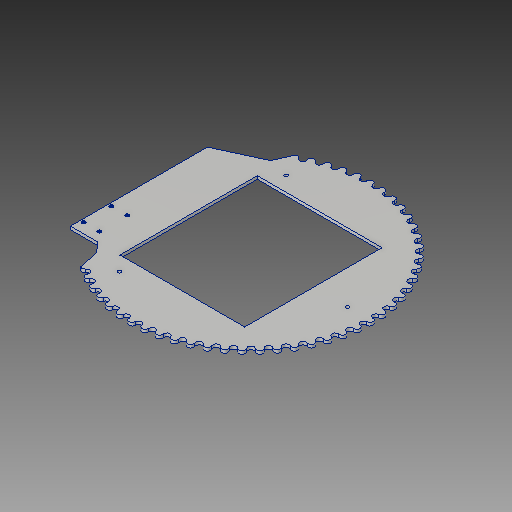
# Autodesk Inventor part: Bearing Plate
Saved by Autodesk Inventor 2019.4 (Build 234330000, 330)
## iProperties
Created: 2020-01-22
Part Number: Bearing Plate
Material: Aluminum 6061
Document SubType Name: Modeling
Designer: admin
Density: 2.7 g/cm^3
Appearance: Aluminum - Flat
Mass: 789.639 g
Surface Area: 1277.98 cm^2
Volume: 292.459 cm^3
Author: admin
Autodesk Inventor part; units mm, degrees
ref_plane "YZ Plane" through (0, 0, 0) normal (1, 0, 0) x (0, 1, 0)
ref_plane "XZ Plane" through (0, 0, 0) normal (0, 1, 0) x (-1, 0, 0)
ref_plane "XY Plane" through (0, 0, 0) normal (0, 0, 1) x (1, 0, 0)
sketch "Sketch1" plane through (0, 0, 0) normal (0, 1, 0) x (-1, 0, 0)
  arc A0 (72.921356, -159.083236) -> (136.106576, 110) centre (0, 0) ccw construction
  circle A1 centre (0, 0) radius 101.6 construction
  line L0 (-100.2, 110.3) -> (100.2, 110.3)
  line L1 (100.2, 110.3) -> (100.2, -110.3)
  line L2 (100.2, -110.3) -> (-100.2, -110.3)
  line L3 (-100.2, -110.3) -> (-100.2, 110.3)
  line L4 (-100.2, 110.3) -> (100.2, -110.3) construction
  line L5 (100.2, 110.3) -> (-100.2, -110.3) construction
  line L6 (180, 110) -> (180, -110)
  line L7 (180, -110) -> (72.921356, -159.083236)
  line L8 (180, 0) -> (0, 0)
  line L9 (180, 110) -> (136.106576, 110)
  arc A2 (136.106576, 110) -> (72.921356, -159.083236) centre (0, 0) ccw
  dimension "d0" = 350
  dimension "d1" = 203.2
  dimension "d4" = 220.6
  dimension "d5" = 200.4
  dimension "d6" = 180
  dimension "d7" = 110
  constraints: 20 end point, 4 point on circle, 3 centre point, 3 midpoint, 2 coincident, 2 horizontal, 2 parallel, 2 perpendicular, 1 tangent, 1 vertical
  measures "d0" diameter of A0
  measures "d1" diameter of A1
  measures "d4" distance of L2.end L0.start
  measures "d5" distance of L0.start L0.end
  measures "d6" distance from line of point (0, 0) L6
  measures "d7" distance from line of point (0, 0) L9
extrude "Extrusion1" add sketch "Sketch1" along normal blind 5
sketch "Sketch2" plane through (0, 0, 0) normal (0, -1, 0) x (1, 0, 0)
  circle A0 centre (-174.837015, 94.1064) radius 2.0193 construction
  circle A1 centre (-174.837015, 49.275) radius 2.0193 construction
  circle A2 centre (-149.437015, 94.1064) radius 2.0193 construction
  circle A3 centre (-149.437015, 49.275) radius 2.0193 construction
  circle A4 centre (-174.837015, 94.1064) radius 3
  circle A5 centre (-149.437015, 94.1064) radius 3
  circle A6 centre (-149.437015, 49.275) radius 3
  circle A7 centre (-174.837015, 49.275) radius 3
  point P0 (0, 0)
  dimension "d8" = 6
  dimension "d9" = 6
  dimension "d10" = 6
  dimension "d11" = 6
  constraints: 4 centre point, 4 coincident
  measures "d8" diameter of A4
  measures "d9" diameter of A5
  measures "d10" diameter of A6
  measures "d11" diameter of A7
extrude "Extrusion2" cut sketch "Sketch2" against normal through all
chamfer "Chamfer1" distance 4 angle 45 4 edges at (-177.837, 0, 49.275) (-152.437, 0, 49.275) (-177.837, 0, 94.1064) (-152.437, 0, 94.1064)
sketch "Sketch3" plane through (0, 5, 0) normal (0, 1, 0) x (1, 0, 0)
  line L0 (154.73, 0) -> (-77.365, -134.000111) construction
  line L1 (-77.365, -134.000111) -> (-77.365, 134.000111) construction
  line L2 (-77.365, 134.000111) -> (154.73, 0) construction
  circle A0 centre (-77.365, 134.000111) radius 2.75
  circle A1 centre (-77.365, -134.000111) radius 2.75
  circle A2 centre (154.73, 0) radius 2.75
  point P0 (0, 0)
  point P1 (0, 0)
  dimension "d17" = 268.00022
  dimension "d18" = 5.5
  dimension "d19" = 5.5
  dimension "d20" = 5.5
  dimension "d23" = 154.73
  constraints: 6 end point, 4 coincident, 3 centre point, 1 vertical, 7 other
  measures "d17" distance of L1.end L0.start
  measures "d18" diameter of A0
  measures "d19" diameter of A1
  measures "d20" diameter of A2
  measures "d23" distance of A2.centre point (0, 0)
extrude "Extrusion3" cut sketch "Sketch3" against normal through all
sketch "Sketch4" plane through (0, 5, 0) normal (0, 1, 0) x (1, 0, 0)
  circle A0 centre (0, 0) radius 191.00775 construction
  arc A1 (190.876865, -4.998287) -> (190.353685, -14.98116) centre (190.745981, -9.996573) ccw
  arc A2 (190.745981, -9.996573) -> (201.00775, 0) centre (191.00775, 0) ccw
  arc A3 (199.906609, -21.011031) -> (190.745981, -9.996573) centre (189.96139, -19.965747) ccw
  line L0 (0, 0) -> (199.906609, -21.011031) construction
  arc A4 (189.308759, -24.922971) -> (193.655834, -29.934348) centre (188.656128, -29.880195) ccw construction
  line L1 (0, 0) -> (201.00775, 0)
  arc A5 (195.744062, 9.858079) -> (190.876865, 4.998287) centre (190.745981, 9.996573) ccw construction
  arc A6 (189.308759, -24.922971) -> (190.353685, -14.98116) centre (189.96139, -19.965747) ccw
  arc A7 (190.876865, -4.998287) -> (190.876865, 4.998287) centre (191.00775, 0) ccw
  arc A8 (-136.106576, -110) -> (-72.921356, 159.083236) centre (0, 0) ccw
  line L2 (196.00775, 0) -> (175, 0)
  line L3 (194.933999, -20.488389) -> (174.041332, -18.292481)
  arc A9 (201.00775, 0) -> (190.745981, 9.996573) centre (191.00775, 0) ccw
  arc A10 (190.745981, 9.996573) -> (199.906609, 21.011031) centre (189.96139, 19.965747) ccw
  arc A11 (199.906609, 21.011031) -> (188.656128, 29.880195) centre (189.96139, 19.965747) ccw
  arc A12 (188.656128, 29.880195) -> (196.615248, 41.791861) centre (186.833772, 39.712744) ccw
  arc A13 (196.615248, 41.791861) -> (184.499319, 49.436443) centre (186.833772, 39.712744) ccw
  arc A14 (184.499319, 49.436443) -> (191.169731, 62.114811) centre (181.659165, 59.024641) ccw
  arc A15 (191.169731, 62.114811) -> (178.321097, 68.451056) centre (181.659165, 59.024641) ccw
  arc A16 (178.321097, 68.451056) -> (183.629717, 81.757217) centre (174.494262, 77.689851) ccw
  arc A17 (183.629717, 81.757217) -> (170.189151, 86.715704) centre (174.494262, 77.689851) ccw
  arc A18 (170.189151, 86.715704) -> (174.077818, 100.503875) centre (165.417564, 95.503875) ccw
  arc A19 (174.077818, 100.503875) -> (160.192578, 104.030277) centre (165.417564, 95.503875) ccw
  arc A20 (160.192578, 104.030277) -> (162.618686, 118.149391) centre (154.528516, 112.271539) ccw
  arc A21 (162.618686, 118.149391) -> (148.440902, 120.205072) centre (154.528516, 112.271539) ccw
  arc A22 (148.440902, 120.205072) -> (149.377869, 134.500438) centre (141.946421, 127.809132) ccw
  arc A23 (149.377869, 134.500438) -> (135.062875, 135.062875) centre (141.946421, 127.809132) ccw
  arc A24 (135.062875, 135.062875) -> (134.500438, 149.377869) centre (127.809132, 141.946421) ccw
  arc A25 (134.500438, 149.377869) -> (120.205072, 148.440902) centre (127.809132, 141.946421) ccw
  arc A26 (120.205072, 148.440902) -> (118.149391, 162.618686) centre (112.271539, 154.528516) ccw
  arc A27 (118.149391, 162.618686) -> (104.030277, 160.192578) centre (112.271539, 154.528516) ccw
  arc A28 (104.030277, 160.192578) -> (100.503875, 174.077818) centre (95.503875, 165.417564) ccw
  arc A29 (100.503875, 174.077818) -> (86.715704, 170.189151) centre (95.503875, 165.417564) ccw
  arc A30 (86.715704, 170.189151) -> (81.757217, 183.629717) centre (77.689851, 174.494262) ccw
  arc A31 (81.757217, 183.629717) -> (68.451056, 178.321097) centre (77.689851, 174.494262) ccw
  arc A32 (68.451056, 178.321097) -> (62.114811, 191.169731) centre (59.024641, 181.659165) ccw
  arc A33 (62.114811, 191.169731) -> (49.436443, 184.499319) centre (59.024641, 181.659165) ccw
  arc A34 (49.436443, 184.499319) -> (41.791861, 196.615248) centre (39.712744, 186.833772) ccw
  arc A35 (41.791861, 196.615248) -> (29.880195, 188.656128) centre (39.712744, 186.833772) ccw
  arc A36 (29.880195, 188.656128) -> (21.011031, 199.906609) centre (19.965747, 189.96139) ccw
  arc A37 (21.011031, 199.906609) -> (9.996573, 190.745981) centre (19.965747, 189.96139) ccw
  arc A38 (9.996573, 190.745981) -> (0, 201.00775) centre (0, 191.00775) ccw
  arc A39 (0, 201.00775) -> (-9.996573, 190.745981) centre (0, 191.00775) ccw
  arc A40 (-9.996573, 190.745981) -> (-21.011031, 199.906609) centre (-19.965747, 189.96139) ccw
  arc A41 (-21.011031, 199.906609) -> (-29.880195, 188.656128) centre (-19.965747, 189.96139) ccw
  arc A42 (-29.880195, 188.656128) -> (-41.791861, 196.615248) centre (-39.712744, 186.833772) ccw
  arc A43 (-41.791861, 196.615248) -> (-49.436443, 184.499319) centre (-39.712744, 186.833772) ccw
  arc A44 (-49.436443, 184.499319) -> (-62.114811, 191.169731) centre (-59.024641, 181.659165) ccw
  arc A45 (-62.114811, 191.169731) -> (-68.451056, 178.321097) centre (-59.024641, 181.659165) ccw
  arc A46 (-68.451056, 178.321097) -> (-81.757217, 183.629717) centre (-77.689851, 174.494262) ccw
  arc A47 (-81.757217, 183.629717) -> (-86.715704, 170.189151) centre (-77.689851, 174.494262) ccw
  arc A48 (-86.715704, 170.189151) -> (-100.503875, 174.077818) centre (-95.503875, 165.417564) ccw
  arc A49 (196.381925, -42.874879) -> (188.488576, -30.919527) centre (186.612056, -40.741883) ccw
  arc A50 (188.488576, -30.919527) -> (199.787769, -22.112505) centre (189.848462, -21.012423) ccw
  arc A51 (190.47343, -64.218284) -> (183.943176, -51.467159) centre (180.997506, -61.023467) ccw
  arc A52 (183.943176, -51.467159) -> (196.142635, -43.956594) centre (186.384672, -41.769783) ccw
  arc A53 (182.252846, -84.782165) -> (177.164955, -71.39005) centre (173.18589, -80.56431) ccw
  arc A54 (177.164955, -71.39005) -> (190.116596, -65.26711) centre (180.658423, -62.020115) ccw
  arc A55 (171.81996, -104.316906) -> (168.236192, -90.446362) centre (163.272033, -99.127211) ccw
  arc A56 (168.236192, -90.446362) -> (181.782798, -85.785371) centre (172.739227, -81.517607) ccw
  arc A57 (159.301412, -122.585382) -> (157.265268, -108.404778) centre (151.376274, -116.486841) ccw
  arc A58 (157.265268, -108.404778) -> (171.242404, -105.262314) centre (162.72321, -100.025585) ccw
  arc A59 (144.84916, -139.365836) -> (144.385358, -125.047307) centre (137.643012, -132.43248) ccw
  arc A60 (144.385358, -125.047307) -> (158.623358, -123.461515) centre (150.731953, -117.319388) ccw
  arc A61 (128.638636, -154.454578) -> (129.752805, -140.171931) centre (122.238951, -146.770567) ccw
  arc A62 (129.752805, -140.171931) -> (144.07884, -140.162061) centre (136.911015, -133.189093) ccw
  arc A63 (110.866614, -167.668451) -> (113.545228, -153.595058) centre (105.351074, -159.327059) ccw
  arc A64 (113.545228, -153.595058) -> (127.7854, -155.161229) centre (121.428163, -147.442063) ccw
  arc A65 (91.74882, -178.847056) -> (95.959367, -165.153748) centre (87.184378, -169.949536) ccw
  arc A66 (95.959367, -165.153748) -> (109.940819, -168.27695) centre (104.471337, -159.905285) ccw
  arc A67 (71.517321, -187.8547) -> (77.208688, -174.707696) centre (67.959382, -178.509056) ccw
  arc A68 (77.208688, -174.707696) -> (90.761704, -179.350017) centre (86.246371, -170.427475) ccw
  arc A69 (50.417698, -194.582043) -> (57.520801, -182.140929) centre (47.909451, -184.901717) ccw
  arc A70 (57.520801, -182.140929) -> (70.480866, -188.246018) centre (66.974491, -178.880905) ccw
  arc A71 (28.706072, -198.947423) -> (37.134689, -187.363218) centre (27.277964, -189.049923) ccw
  arc A72 (37.134689, -187.363218) -> (49.344485, -194.856966) centre (46.889631, -185.162964) ccw
  arc A73 (6.645993, -200.897851) -> (16.297812, -190.311171) centre (6.31536, -190.903318) ccw
  arc A74 (16.297812, -190.311171) -> (27.60913, -199.102616) centre (26.235594, -189.197395) ccw
  arc A75 (-15.494758, -200.409651) -> (-4.736898, -190.949005) centre (-14.723905, -190.439406) ccw
  arc A76 (-4.736898, -190.949005) -> (5.538636, -200.931429) centre (5.263093, -190.935226) ccw
  arc A77 (-37.447425, -197.488749) -> (-25.714108, -189.268976) centre (-35.584441, -187.663817) ccw
  arc A78 (-25.714108, -189.268976) -> (-16.599088, -200.321207) centre (-15.773295, -190.355362) ccw
  arc A79 (-58.94553, -192.170601) -> (-46.379184, -185.291478) centre (-56.01303, -182.610244) ccw
  arc A80 (-46.379184, -185.291478) -> (-38.535323, -197.279356) centre (-36.618216, -187.464842) ccw
  arc A81 (-79.728117, -184.519763) -> (-66.48128, -179.064793) centre (-75.761697, -175.340029) ccw
  arc A82 (-66.48128, -179.064793) -> (-60.003791, -191.842802) centre (-57.018642, -182.298752) ccw
  arc A83 (-99.542912, -174.629105) -> (-85.776383, -170.664503) centre (-94.590719, -165.941425) ccw
  arc A84 (-85.776383, -170.664503) -> (-80.743894, -184.077536) centre (-76.726939, -174.919803) ccw
  arc A85 (-118.149391, -162.618686) -> (-104.030277, -160.192578) centre (-112.271539, -154.528516) ccw
  arc A86 (-104.030277, -160.192578) -> (-100.503875, -174.077818) centre (-95.503875, -165.417564) ccw
  dimension "d24" = 5
  dimension "d28" = 5
  dimension "d30" = 6
  dimension "d31" = 5
  dimension "d32" = 5
  dimension "d33" = 5
  dimension "d45" = 120
  dimension "d49" = 120
  constraints: 179 point on circle, 86 centre point, 8 end point, 4 equal radius, 4 point on line, 3 coincident, 1 horizontal, 275 other
  measures "d24" radius of A1
  measures "d28" radius of A4
  measures "d30" angle of L0 L1
  measures "d31" radius of A5
  measures "d32" radius of A6
  measures "d33" radius of A7
extrude "Extrusion4" add sketch "Sketch4" against normal up to surface (5 mm away)
pattern_circular "Circular Pattern1" count 41 over 240 about axis through (0, -10, 0) along (0, 1, 0) of "Extrusion4" both ways yes
sketch "Sketch5" plane through (0, 5, 0) normal (0, 1, 0) x (1, 0, 0)
  line L0 (-115.210465, -158.573601) -> (-122.032817, -125.431223)
  arc A0 (-91.109789, 167.803358) -> (-98.003875, 169.747691) centre (-95.503875, 165.417564) ccw
  line L1 (-98.003875, 169.747691) -> (-110.712806, 141.760205)
  line L2 (-87.886297, 152.223532) -> (-180, 110)
  line L3 (-87.886297, 152.223532) -> (-98.003875, 169.747691)
  arc A1 (-136.106576, -110) -> (-102.862419, -141.577974) centre (0, 0) ccw
  line L4 (-115.210465, -158.573601) -> (-102.862419, -141.577974)
  dimension "d51" = 25
  dimension "d52" = 25
  constraints: 6 end point, 1 point on circle, 1 point on line
  measures "d51" distance from line of L4 L0.end
  measures "d52" distance from line of L3 L1.end
extrude "Extrusion5" add sketch "Sketch5" against normal up to surface (5 mm away)
body "Solid1"
